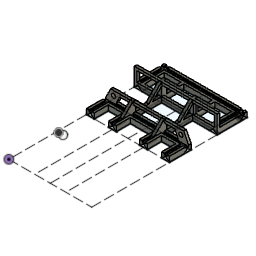
Body (1) (Autodesk Fusion 360 design; units mm, degrees)
Autodesk Fusion 360 part; units mm, degrees
sketch "스케치1" plane through (0, 0, 0) normal (0, 0, 1) x (1, 0, 0)
  line L0 (0, 0) -> (160, 0) construction
  line L1 (160, 0) -> (160, 300) construction
  line L2 (160, 300) -> (0, 300) construction
  line L3 (0, 300) -> (0, 0) construction
  line L4 (80, 0) -> (80, 300) construction
  line L5 (160, 150) -> (0, 150) construction
  line L6 (0, 192.1) -> (47.5, 192.1)
  line L7 (47.5, 192.1) -> (47.5, 242.1)
  line L8 (47.5, 242.1) -> (0, 242.1)
  line L9 (0, 242.1) -> (0, 300)
  line L10 (0, 300) -> (160, 300)
  line L11 (160, 300) -> (160, 242.1)
  line L12 (160, 242.1) -> (112.5, 242.1)
  line L13 (112.5, 242.1) -> (112.5, 192.1)
  line L14 (112.5, 192.1) -> (160, 192.1)
  line L15 (52.5, 242.1) -> (107.5, 242.1)
  line L16 (107.5, 242.1) -> (107.5, 192.1)
  line L17 (107.5, 192.1) -> (52.5, 192.1)
  line L18 (52.5, 192.1) -> (52.5, 242.1)
  line L19 (0, 247.1) -> (160, 247.1) construction
  line L20 (50, 300) -> (50, 0) construction
  line L21 (110, 300) -> (110, 0) construction
  line L22 (0, 97.8296) -> (15, 97.8296)
  line L23 (15, 97.8296) -> (15, 87.8296)
  line L24 (15, 87.8296) -> (0, 87.8296)
  line L25 (0, 87.8296) -> (0, 97.8296)
  circle A0 centre (3.4, 92.8296) radius 2
  circle A1 centre (3.4, 92.8296) radius 3.4 construction
  line L26 (6.8, 94.7926) -> (6.8, 90.8666)
  line L27 (6.8, 90.8666) -> (3.4, 88.9036)
  line L28 (3.4, 88.9036) -> (0, 90.8666)
  line L29 (0, 90.8666) -> (0, 94.7926)
  line L30 (0, 94.7926) -> (3.4, 96.7556)
  line L31 (3.4, 96.7556) -> (6.8, 94.7926)
  line L32 (0, 92.8296) -> (15, 92.8296) construction
  line L33 (15, 94.7926) -> (15, 90.8666)
  circle A2 centre (11.6, 92.8296) radius 2
  line L34 (11.6, 96.7556) -> (15, 94.7926)
  line L35 (15, 90.8666) -> (11.6, 88.9036)
  line L36 (11.6, 88.9036) -> (8.2, 90.8666)
  line L37 (8.2, 94.7926) -> (11.6, 96.7556)
  circle A3 centre (11.6, 92.8296) radius 3.4 construction
  line L38 (8.2, 90.8666) -> (8.2, 94.7926)
  line L39 (7.5, 97.8296) -> (7.5, 87.8296) construction
  line L40 (15, 242.1) -> (15, 285)
  line L41 (15, 285) -> (145, 285)
  line L42 (145, 285) -> (145, 242.1)
  line L43 (160, 247.1) -> (0, 247.1)
  line L44 (160, 192.1) -> (160, 150)
  line L45 (160, 150) -> (145, 150)
  line L46 (145, 150) -> (145, 177.1)
  line L47 (145, 177.1) -> (117.5, 177.1)
  line L48 (117.5, 177.1) -> (117.5, 150)
  line L49 (117.5, 150) -> (102.5, 150)
  line L50 (102.5, 150) -> (102.5, 177.1)
  line L51 (102.5, 177.1) -> (57.5, 177.1)
  line L52 (57.5, 177.1) -> (57.5, 150)
  line L53 (57.5, 150) -> (42.5, 150)
  line L54 (42.5, 150) -> (42.5, 177.1)
  line L55 (42.5, 177.1) -> (15, 177.1)
  line L56 (15, 177.1) -> (15, 150)
  line L57 (15, 150) -> (0, 150)
  line L58 (0, 150) -> (0, 192.1)
  circle A4 centre (152.5, 292.5) radius 1.5
  circle A5 centre (142.5, 292.5) radius 1.5
  line L59 (152.5, 291) -> (142.5, 291)
  line L60 (142.5, 294) -> (152.5, 294)
  line L61 (152.5, 292.5) -> (142.5, 292.5) construction
  dimension "d1" = 300
  dimension "d2" = 160
  dimension "d16" = 50
  dimension "d48" = 5
  dimension "d51" = 5
  dimension "d52" = 60
  dimension "d83" = 57.9
  dimension "d93" = 10
  dimension "d97" = 15
  dimension "d98" = 4
  dimension "d99" = 6.8
  dimension "d100" = 120
  dimension "d101" = 120
  dimension "d102" = 4
  dimension "d103" = 6.8
  dimension "d104" = 120
  dimension "d105" = 120
  dimension "d106" = 3.4
  dimension "d137" = 15
  dimension "d138" = 15
  dimension "d139" = 15
  dimension "d146" = 15
  dimension "d147" = 15
  dimension "d148" = 15
  dimension "d193" = 3
  dimension "d194" = 3
  dimension "d196" = 10
  dimension "d199" = 7.5
  dimension "d200" = 7.5
  constraint coincident L0.start L3.end
  constraint horizontal L0
  constraint perpendicular L0 L1
  constraint perpendicular L1 L2
  constraint perpendicular L0 L3
  constraint midpoint L0 L4.start
  constraint midpoint L2 L4.end
  constraint midpoint L1 L5.start
  constraint midpoint L3 L5.end
  constraint coincident L3 L6.start
  constraint perpendicular L6 L7
  constraint coincident L3 L8.end
  constraint perpendicular L3 L8
  constraint coincident L1 L11.end
  constraint perpendicular L1 L12
  constraint perpendicular L12 L13
  constraint coincident L1 L14.end
  constraint perpendicular L1 L14
  constraint symmetric L4 L7 L13
  constraint symmetric L4 L8 L12
  constraint symmetric L4 L6 L14
  constraint horizontal L15
  constraint vertical L16
  constraint horizontal L17
  constraint vertical L18
  constraint symmetric L4 L16 L18
  constraint coincident L3 L19.start
  constraint coincident L11 L19.end
  constraint horizontal L19
  constraint coincident L10 L20.start
  constraint coincident L0 L20.end
  constraint vertical L20
  constraint symmetric L7 L18 L20
  constraint coincident L10 L21.start
  constraint coincident L0 L21.end
  constraint perpendicular L0 L21
  constraint symmetric L13 L16 L21
  constraint collinear L12 L15
  constraint collinear L14 L17
  constraint horizontal L22
  constraint vertical L23
  constraint horizontal L24
  constraint vertical L25
  constraint coincident L3 L22.start
  constraint concentric A0 A1
  constraint vertical L26
  constraint tangent A1 L26
  constraint tangent A1 L31
  constraint tangent A1 L30
  constraint tangent A1 L27
  constraint tangent A1 L28
  constraint tangent A1 L29
  constraint vertical L29
  constraint parallel L27 L30
  constraint parallel L28 L31
  constraint midpoint L25 L32.start
  constraint midpoint L23 L32.end
  constraint concentric A2 A3
  constraint vertical L33
  constraint tangent L33 A3
  constraint tangent L34 A3
  constraint tangent L37 A3
  constraint tangent L35 A3
  constraint tangent L36 A3
  constraint tangent A3 L38
  constraint vertical L38
  constraint parallel L35 L37
  constraint parallel L34 L36
  constraint coincident A0.centre L32
  constraint midpoint L22 L39.start
  constraint midpoint L24 L39.end
  constraint symmetric A0.centre A2.centre L39
  constraint coincident L8 L40.start
  constraint perpendicular L8 L40
  constraint perpendicular L40 L41
  constraint coincident L12 L42.end
  constraint perpendicular L12 L42
  constraint coincident L5 L45.end
  constraint perpendicular L44 L45
  constraint perpendicular L45 L46
  constraint perpendicular L46 L47
  constraint coincident L5 L48.end
  constraint perpendicular L5 L48
  constraint coincident L5 L49.end
  constraint perpendicular L49 L50
  constraint perpendicular L50 L51
  constraint coincident L5 L52.end
  constraint perpendicular L5 L52
  constraint coincident L5 L53.end
  constraint perpendicular L5 L54
  constraint perpendicular L54 L55
  constraint coincident L5 L56.end
  constraint perpendicular L5 L56
  constraint perpendicular L3 L57
  constraint symmetric L20 L52 L54
  constraint symmetric L21 L48 L50
  constraint symmetric L4 L50 L52
  constraint collinear L47 L51
  constraint collinear L51 L55
  constraint coincident A4 L59.start
  constraint coincident A5 L59.end
  constraint tangent A5 L59
  constraint coincident A5 L60.start
  constraint coincident A4 L60.end
  constraint tangent A4 L60
  constraint coincident A4.centre L61.start
  constraint coincident A5.centre L61.end
  constraint parallel L59 L61
  constraint parallel L60 L61
  constraint horizontal L61
  measures "d1" distance of L0.end L1.end
  measures "d2" distance of L1.end L2.end
  measures "d16" distance of L6.end L7.end
  measures "d48" distance of L8 L19
  measures "d51" distance of L7 L18
  measures "d52" distance of L20 L21
  measures "d83" distance of L2 L8
  measures "d93" distance of L22.end L23.end
  measures "d97" distance of L22.start L22.end
  measures "d98" diameter of A0
  measures "d99" diameter of A1
  measures "d100" angle of L29 L30
  measures "d101" angle of L26 L31
  measures "d102" diameter of A2
  measures "d103" diameter of A3
  measures "d104" angle of L37 L38
  measures "d105" angle of L33 L34
  measures "d106" distance of L3 A0.centre
  measures "d137" distance of L2 L41
  measures "d138" distance of L1 L42
  measures "d139" distance of L3 L40
  measures "d146" distance of L1 L46
  measures "d147" distance of L14 L47
  measures "d148" distance of L48 L50
  measures "d193" diameter of A5
  measures "d194" diameter of A4
  measures "d196" horizontal distance of A4.centre A5.centre
  measures "d199" distance of L10 L61
  measures "d200" distance of L1 A4.centre
sketch "스케치2" plane through (0, 0, 0) normal (0, 1, 0) x (1, 0, 0)
  line L0 (0, 0) -> (160, 0)
  line L1 (160, 0) -> (160, -10)
  line L2 (160, -10) -> (150.5845, -29)
  line L3 (9.4155, -29) -> (0, -10)
  line L4 (0, -10) -> (0, 0)
  line L5 (0, -118.8837) -> (160, -118.8837) construction
  line L6 (160, -118.8837) -> (160, -153.5837)
  line L7 (160, -153.5837) -> (0, -153.5837)
  line L8 (0, -153.5837) -> (0, -118.8837)
  line L9 (80, 0) -> (80, -153.5837) construction
  line L10 (50, -153.5837) -> (50, 0) construction
  line L11 (110, -153.5837) -> (110, 0) construction
  line L12 (5, -148.5837) -> (45.7, -148.5837)
  line L13 (45.7, -148.5837) -> (45.7, -128.8837)
  line L14 (45.7, -128.8837) -> (5, -128.8837)
  line L15 (5, -128.8837) -> (5, -148.5837)
  line L16 (114.3, -148.5837) -> (155, -148.5837)
  line L17 (155, -148.5837) -> (155, -128.8837)
  line L18 (155, -128.8837) -> (114.3, -128.8837)
  line L19 (114.3, -128.8837) -> (114.3, -148.5837)
  circle A0 centre (145, -138.8837) radius 1.5
  circle A1 centre (15, -138.8837) radius 1.5
  circle A2 centre (15, -20) radius 4
  circle A3 centre (145, -20) radius 4
  line L20 (15, -138.8837) -> (15, -20) construction
  line L21 (145, -138.8837) -> (145, -20) construction
  line L22 (9.4155, -29) -> (150.5845, -29)
  line L23 (27.0267, -24) -> (47.5, -24)
  line L24 (47.5, -24) -> (47.5, -10)
  line L25 (47.5, -10) -> (20.0889, -10)
  line L26 (20.0889, -10) -> (27.0267, -24)
  line L27 (112.5, -24) -> (112.5, -10)
  line L28 (112.5, -10) -> (139.9111, -10)
  line L29 (139.9111, -10) -> (132.9733, -24)
  line L30 (132.9733, -24) -> (112.5, -24)
  line L31 (52.5, -24) -> (107.5, -24)
  line L32 (107.5, -24) -> (107.5, -10)
  line L33 (107.5, -10) -> (52.5, -10)
  line L34 (52.5, -10) -> (52.5, -24)
  line L35 (52.5, -148.5837) -> (107.5, -148.5837)
  line L36 (107.5, -148.5837) -> (107.5, -128.8837)
  line L37 (107.5, -128.8837) -> (52.5, -128.8837)
  line L38 (52.5, -128.8837) -> (52.5, -148.5837)
  line L39 (0, 0) -> (160, 0)
  line L40 (160, -118.8837) -> (158.5, -118.8837)
  line L41 (158.5, -118.8837) -> (152.5, -124.8837)
  line L42 (152.5, -124.8837) -> (146.5, -118.8837)
  line L43 (152.5, -124.8837) -> (152.5, -122.5068) construction
  line L44 (0, -118.8837) -> (1.5, -118.8837)
  line L45 (1.5, -118.8837) -> (7.5, -124.8837)
  line L46 (7.5, -124.8837) -> (13.5, -118.8837)
  line L47 (13.5, -118.8837) -> (146.5, -118.8837)
  line L48 (145, -20) -> (15, -20)
  circle A4 centre (15, -20) radius 1.5
  circle A5 centre (145, -20) radius 1.5
  dimension "d50" = 160
  dimension "d53" = 60
  dimension "d54" = 10
  dimension "d58" = 5
  dimension "d59" = 5
  dimension "d61" = 3
  dimension "d69" = 10
  dimension "d70" = 10
  dimension "d71" = 40.7
  dimension "d72" = 19.7
  dimension "d73" = 10
  dimension "d74" = 8
  dimension "d75" = 20
  dimension "d76" = 9
  dimension "d77" = 9
  dimension "d78" = 5
  dimension "d79" = 9
  dimension "d80" = 5
  dimension "d82" = 10
  dimension "d133" = 45
  dimension "d134" = 1.5
  dimension "d136" = 7.5
  dimension "d145" = 3
  constraint coincident L0.start L4.end
  constraint horizontal L0
  constraint perpendicular L0 L1
  constraint perpendicular L4 L5
  constraint perpendicular L5 L6
  constraint perpendicular L6 L7
  constraint perpendicular L5 L8
  constraint collinear L4 L8
  constraint collinear L1 L6
  constraint midpoint L0 L9.start
  constraint midpoint L7 L9.end
  constraint coincident L7 L10.start
  constraint coincident L0 L10.end
  constraint coincident L7 L11.start
  constraint coincident L0 L11.end
  constraint perpendicular L0 L11
  constraint symmetric L2 L3 L9
  constraint horizontal L12
  constraint vertical L13
  constraint horizontal L14
  constraint vertical L15
  constraint horizontal L16
  constraint vertical L17
  constraint horizontal L18
  constraint vertical L19
  constraint symmetric L9 L13 L19
  constraint symmetric L9 L15 L17
  constraint collinear L12 L16
  constraint collinear L14 L18
  constraint symmetric L9 A0 A1
  constraint symmetric L9 A2 A3
  constraint coincident A1.centre L20.start
  constraint coincident A2.centre L20.end
  constraint coincident A0.centre L21.start
  constraint coincident A3.centre L21.end
  constraint vertical L21
  constraint perpendicular L20 L22
  constraint perpendicular L10 L23
  constraint perpendicular L23 L24
  constraint perpendicular L10 L25
  constraint perpendicular L23 L27
  constraint perpendicular L27 L28
  constraint perpendicular L27 L30
  constraint perpendicular L9 L31
  constraint perpendicular L31 L32
  constraint perpendicular L9 L33
  constraint vertical L34
  constraint parallel L3 L26
  constraint collinear L23 L31
  constraint collinear L30 L31
  constraint collinear L28 L33
  constraint collinear L25 L33
  constraint symmetric L9 L26 L29
  constraint symmetric L9 L24 L27
  constraint symmetric L11 L27 L32
  constraint perpendicular L9 L35
  constraint perpendicular L7 L36
  constraint perpendicular L36 L37
  constraint vertical L38
  constraint collinear L34 L38
  constraint collinear L32 L36
  constraint collinear L18 L37
  constraint collinear L16 L35
  constraint coincident L5 L40.end
  constraint coincident L5 L42.end
  constraint perpendicular L41 L42
  constraint vertical L43
  constraint coincident L5 L44.end
  constraint coincident L5 L46.end
  constraint perpendicular L45 L46
  constraint symmetric L9 L41 L45
  constraint symmetric L9 L42 L46
  constraint equal A4 A5
  measures "d50" distance of L0.start L0.end
  measures "d53" distance of L10 L11
  measures "d54" distance of L3.end L0.start
  measures "d58" distance of L8 L15
  measures "d59" distance of L7 L12
  measures "d61" diameter of A0
  measures "d69" distance of L17 A0.centre
  measures "d70" distance of L18 A0.centre
  measures "d71" distance of L12.start L12.end
  measures "d72" distance of L12.start L14.end
  measures "d73" distance of L5 L14
  measures "d74" diameter of A2
  measures "d75" distance of L0 A2.centre
  measures "d76" distance of A2.centre L22
  measures "d77" distance of L3 A2.centre
  measures "d78" distance of L22 L31
  measures "d79" distance of A2.centre L26
  measures "d80" distance of L27 L32
  measures "d82" distance of L33 L39
  measures "d133" angle of L5 L41
  measures "d134" distance of L5.end L40.end
  measures "d136" distance of L6 L43
  measures "d145" diameter of A4
sketch "스케치4" plane through (0, 0, 0) normal (1, 0, 0) x (0, 1, 0)
  line L0 (0, 0) -> (300, 0) construction
  line L1 (150, 0) -> (150, 280) construction
  line L2 (300, 0) -> (300, 10)
  line L3 (242.1, 0) -> (242.1, 34.7)
  line L4 (242.1, 34.7) -> (252.1, 34.7)
  line L5 (192.1, 0) -> (192.1, 29.6923)
  line L6 (150, 10) -> (150, 0)
  line L7 (300, 10) -> (150, 10) construction
  line L8 (192.1, 0) -> (150, 0)
  line L9 (252.1, 34.7) -> (276.8, 10)
  line L10 (269.7289, 10) -> (252.1, 10)
  line L11 (252.1, 10) -> (252.1, 27.6289)
  line L12 (252.1, 27.6289) -> (269.7289, 10)
  line L13 (167.5749, 10) -> (187.1, 29.6923)
  line L14 (187.1, 29.6923) -> (192.1, 29.6923)
  line L15 (242.1, 34.7) -> (217.4, 10)
  line L16 (192.1, 29.6923) -> (211.7923, 10)
  line L17 (224.4711, 10) -> (242.1, 27.6289)
  line L18 (192.1, 22.6212) -> (204.7212, 10)
  line L19 (242.1, 10) -> (192.1, 10)
  line L20 (300, 0) -> (298.5, 0)
  line L21 (298.5, 0) -> (292.5, 6)
  line L22 (292.5, 6) -> (286.5, 0)
  line L23 (286.5, 0) -> (242.1, 0)
  line L24 (300, 10) -> (295.2, 10)
  line L25 (295.2, 10) -> (295.2, 7.5)
  line L26 (295.2, 7.5) -> (289.8, 7.5)
  line L27 (289.8, 7.5) -> (289.8, 10)
  line L28 (289.8, 10) -> (276.8, 10)
  line L29 (292.5, 7.5) -> (292.5, 6) construction
  line L30 (242.1, 0) -> (192.1, 0)
  line L31 (70, 135) -> (82, 135)
  line L32 (82, 135) -> (76, 141)
  line L33 (76, 141) -> (70, 135)
  line L34 (75.6, 152.5) -> (81, 152.5)
  line L35 (81, 152.5) -> (81, 155)
  line L36 (81, 155) -> (75.6, 155)
  line L37 (75.6, 155) -> (75.6, 152.5)
  line L38 (286.5, 0) -> (298.5, 0)
  line L39 (289.8, 10) -> (295.2, 10)
  line L40 (150, 7.5) -> (165.0749, 7.5)
  line L41 (165.0749, 7.5) -> (167.5749, 10)
  dimension "d111" = 300
  dimension "d112" = 57.9
  dimension "d113" = 50
  dimension "d115" = 34.7
  dimension "d116" = 10
  dimension "d121" = 10
  dimension "d122" = 135
  dimension "d123" = 10
  dimension "d124" = 5
  dimension "d126" = 5
  dimension "d129" = 45
  dimension "d130" = 45
  dimension "d131" = 5
  dimension "d132" = 5
  dimension "d140" = 45
  dimension "d141" = 1.5
  dimension "d142" = 7.5
  dimension "d143" = 2.5
  dimension "d144" = 5.4
  dimension "d157" = 12
  dimension "d158" = 45
  dimension "d159" = 45
  dimension "d160" = 5.4
  dimension "d161" = 2.5
  dimension "d181" = 2.5
  dimension "d184" = 135
  constraint coincident L0.start origin
  constraint horizontal L0
  constraint midpoint L0 L1.start
  constraint perpendicular L0 L1
  constraint perpendicular L0 L2
  constraint coincident L0 L3.start
  constraint perpendicular L0 L3
  constraint coincident L0 L5.start
  constraint perpendicular L0 L5
  constraint coincident L0 L1.start
  constraint perpendicular L0 L6
  constraint horizontal L4
  constraint coincident L1 L6.start
  constraint perpendicular L1 L7
  constraint coincident L7 L9.end
  constraint coincident L7 L10.start
  constraint coincident L7 L10.end
  constraint perpendicular L10 L11
  constraint parallel L9 L12
  constraint coincident L6.start L7
  constraint coincident L7 L13.start
  constraint horizontal L14
  constraint coincident L7 L15.end
  constraint coincident L7 L16.end
  constraint coincident L7 L17.start
  constraint coincident L3 L17.end
  constraint parallel L15 L17
  constraint coincident L5 L18.start
  constraint coincident L7 L18.end
  constraint perpendicular L17 L18
  constraint coincident L7 L19.start
  constraint coincident L3 L19.start
  constraint coincident L7 L19.end
  constraint coincident L5 L19.end
  constraint coincident L0 L20.end
  constraint coincident L0 L22.end
  constraint perpendicular L21 L22
  constraint coincident L7 L24.end
  constraint perpendicular L7 L25
  constraint perpendicular L25 L26
  constraint coincident L7 L27.end
  constraint perpendicular L7 L27
  constraint midpoint L26 L29.start
  constraint vertical L29
  constraint collinear L1 L6
  constraint horizontal L31
  constraint parallel L31 L34
  constraint perpendicular L31 L35
  constraint perpendicular L35 L36
  constraint perpendicular L36 L37
  constraint coincident L6 L40.start
  constraint perpendicular L6 L40
  measures "d111" distance of L0.start L0.end
  measures "d112" distance of L2 L3
  measures "d113" distance of L3 L5
  measures "d115" distance of L3.start L3.end
  measures "d116" distance of L0.end L2.end
  measures "d121" distance of L4.end L3.end
  measures "d122" angle of L7 L9
  measures "d123" distance of L3 L11
  measures "d124" distance of L9 L12
  measures "d126" distance of L5.end L13.end
  measures "d129" angle of L5 L16
  measures "d130" angle of L3 L15
  measures "d131" distance of L16 L18
  measures "d132" distance of L15 L17
  measures "d140" angle of L0 L21
  measures "d141" distance of L0.end L20.end
  measures "d142" distance of L2 L29
  measures "d143" distance of L24.end L25.end
  measures "d144" distance of L25.end L26.end
  measures "d157" distance of L31.start L31.end
  measures "d158" angle of L31 L32
  measures "d159" angle of L31 L33
  measures "d160" distance of L35.end L36.end
  measures "d161" distance of L34.end L35.end
  measures "d181" distance of L7 L40
  measures "d184" angle of L40 L41
extrude "돌출1" add sketch "스케치1" along normal blind 10 contours L6 L7 L8 L12 L13 L14 L40 L42 L43 L44 L45 L46 L47 L48 L49 L50 L51 L52 L53 L54 L55 L56 L57 L58 | L8 L9 L40 L43 | L9 L10 L11 L40 L41 L42 L43 | L11 L12 L42 L43 | A4 | A4 A5 L59 L60 | A5 makes body 1
extrude "돌출5" add sketch "스케치4" along normal blind 350 separate body contours L31 L32 L33 makes body 2
move_body "정렬5" bodies 2 to x (1, 0, 0) y (0, 1, 0) z (0, 0, 1) at (0, 110.1, -135)
move_body "이동2" bodies 2 to x (1, 0, 0) y (0, 1, 0) z (0, 0, 1) at (0, -1.5, 0)
combine "결합5" operation cut target body 1 tool bodies 2
extrude "돌출6" cut sketch "스케치4" along normal blind 200 contours L21 L22 L38 bodies 1
extrude "돌출7" cut sketch "스케치4" along normal blind 180 contours L25 L26 L27 L39 bodies 1
extrude "돌출8" add sketch "스케치4" along normal blind 290 separate body contours L34 L35 L36 L37 makes body 3
move_body "정렬6" bodies 3 to x (1, 0, 0) y (0, 1, 0) z (0, 0, 1) at (-130, 111.1, -145)
move_body "이동3" bodies 3 to x (1, 0, 0) y (0, 1, 0) z (0, 0, 1) at (0, -4.8, 0)
combine "결합6" operation cut target body 1 tool bodies 3
extrude "돌출9" add sketch "스케치4" along normal blind 250 separate body contours L31 L32 L33 makes body 4
move_body "정렬7" bodies 4 to x (0, 1, 0) y (-1, 0, 0) z (0, 0, 1) at (83.5, 150, -135)
combine "결합7" operation cut target body 1 tool bodies 4
extrude "돌출10" add sketch "스케치4" along normal blind 240 separate body contours L34 L35 L36 L37 makes body 5
move_body "정렬8" bodies 5 to x (0, 1, 0) y (-1, 0, 0) z (0, 0, 1) at (85.8, 150, -145)
combine "결합8" operation cut target body 1 tool bodies 5
extrude "돌출11" add sketch "스케치4" along normal blind 34.6 separate body contours L31 L32 L33 | L34 L35 L36 L37 makes body 6 at (23.0667, 74, 135) makes body 7 at (11.5333, 79.2, 155)
move_body "정렬9" bodies 6 to x (0, 1, 0) y (-1, 0, 0) z (0, 0, 1) at (126, 150, -135)
combine "결합9" operation cut target body 1 tool bodies 6
move_body "정렬10" bodies 7 to x (0, 1, 0) y (-1, 0, 0) z (0, 0, 1) at (128.3, 150, -145)
combine "결합10" operation cut target body 1 tool bodies 7
extrude "돌출12" add sketch "스케치4" along normal blind 34.6 separate body contours L31 L32 L33 | L34 L35 L36 L37 makes body 8 at (23.0667, 74, 135) makes body 9 at (11.5333, 79.2, 155)
move_body "정렬11" bodies 8 to x (0, 1, 0) y (-1, 0, 0) z (0, 0, 1) at (186, 150, -135)
move_body "정렬12" bodies 9 to x (0, 1, 0) y (-1, 0, 0) z (0, 0, 1) at (188.3, 150, -145)
combine "결합11" operation cut target body 1 tool bodies 8
combine "결합12" operation cut target body 1 tool bodies 9
extrude "돌출13" add sketch "스케치4" along normal blind 250 separate body contours L31 L32 L33 | L34 L35 L36 L37 makes body 10 at (83.3333, 79.2, 155) makes body 11 at (83.3333, 74, 135)
move_body "정렬13" bodies 10 to x (0, 1, 0) y (-1, 0, 0) z (0, 0, 1) at (230.8, 150, -145)
move_body "정렬14" bodies 11 to x (0, 1, 0) y (-1, 0, 0) z (0, 0, 1) at (228.5, 150, -135)
combine "결합13" operation cut target body 1 tool bodies 10
combine "결합14" operation cut target body 1 tool bodies 11
extrude "돌출14" add sketch "스케치4" along normal blind 5.4 separate body contours L2 L3 L4 L9 L20 L21 L22 L23 L24 L25 L26 L27 L28 | L3 L5 L19 L30 | L5 L6 L8 L13 L14 L40 L41 | L3 L15 L17 L19 | L5 L16 L18 L19 makes body 12
copy_body "CopyPasteBodies2" bodies 12 makes body 13
move_body "이동4" bodies 13 to x (1, 0, 0) y (0, 1, 0) z (0, 0, 1) at (60, 0, 0)
move_body "정렬15" bodies 12 to x (1, 0, 0) y (0, 1, 0) z (0, 0, 1) at (47.3, 0, 0)
move_body "정렬16" bodies 13 to x (1, 0, 0) y (0, 1, 0) z (0, 0, 1) at (47.3, 0, 0)
combine "결합15" operation add target body 13 tool bodies 1
combine "결합16" operation add target body 12 tool bodies 13
extrude "돌출15" add sketch "스케치2" along normal blind 5 separate body contours L6 L7 L8 L40 L41 L42 L44 L45 L46 L47 makes body 14
move_body "정렬17" bodies 14 to x (1, 0, 0) y (0, 1, 0) z (0, 0, 1) at (0, 242.1, -118.8837)
extrude "돌출16" add sketch "스케치2" along normal blind 5 separate body contours L0 L1 L2 L3 L4 L22 L39 makes body 15
move_body "정렬18" bodies 15 to x (1, 0, 0) y (0, 1, 0) z (0, 0, 1) at (0, 187.1, 0)
combine "결합17" operation add target body 14 tool bodies 12
combine "결합18" operation add target body 14 tool bodies 15
extrude "돌출17" add sketch "스케치4" along normal blind 34.6 separate body contours L31 L32 L33 makes body 16
copy_body "CopyPasteBodies3" bodies 16 makes body 17
move_body "이동5" bodies 17 to x (1, 0, 0) y (0, 1, 0) z (0, 0, 1) at (0, 25, 0)
move_body "정렬19" bodies 17 to x (0, -1, 0) y (1, 0, 0) z (0, 0, 1) at (-51, 184.6, -135)
move_body "정렬20" bodies 16 to x (0, -1, 0) y (1, 0, 0) z (0, 0, 1) at (34, 184.6, -135)
combine "결합19" operation cut target body 14 tool bodies 16
combine "결합20" operation cut target body 14 tool bodies 17
extrude "돌출18" add sketch "스케치4" along normal blind 180 separate body contours L31 L32 L33 makes body 18
move_body "정렬21" bodies 18 to x (1, 0, 0) y (0, 1, 0) z (0, 0, 1) at (0, 108.6, -135)
combine "결합21" operation cut target body 14 tool bodies 18
extrude "돌출19" add sketch "스케치1" along normal blind 10 separate body contours A4 | A4 A5 L59 L60 | A5 makes body 19
pattern_linear "R-패턴2" count 7 spacing 20 along (-1, 0, 0) of bodies 19 makes body 20 at (125.8333, 294, 3.3333) makes body 21 at (105.8333, 294, 3.3333) makes body 22 at (85.8333, 294, 3.3333) makes body 23 at (65.8333, 294, 3.3333) makes body 24 at (45.8333, 294, 3.3333) makes body 25 at (25.8333, 294, 3.3333)
combine "결합23" operation cut target body 14 tool bodies 19
combine "결합24" operation cut target body 14 tool bodies 20
combine "결합25" operation cut target body 14 tool bodies 21
combine "결합26" operation cut target body 14 tool bodies 22
combine "결합27" operation cut target body 14 tool bodies 23
combine "결합28" operation cut target body 14 tool bodies 24
equation "m3hole = 3 mm" comment "m3 볼트 스크류 크기"
equation "m3width = 5.4 mm" comment "m3너트 크기"
equation "m3height = 2.5 mm" comment "m3너트 높이"
equation "frame = 15 mm" comment "레일 너비"
equation "thk = 10 mm" comment "뼈대 너비"
equation "thn = 5 mm"
equation "error = 0.4 mm" comment "공차"
equation "d48 = thn"
equation "d50 = d2"
equation "d51 = thn"
equation "d53 = d52"
equation "d54 = thk"
equation "d58 = thn"
equation "d59 = thn"
equation "bearing_height = 4 mm"
equation "bearing_out = 8 mm" comment "베어링 밖쪽 반지름"
equation "bearing_in = 3 mm" comment "베어링 안쪽 반지름"
equation "moter_len = 19.7 mm"
equation "moter_wid = 40.7 mm"
equation "moter_hole_len = 10 mm"
equation "moter_hole_wid = 10 mm"
equation "d69 = moter_hole_wid"
equation "d70 = moter_hole_len"
equation "d71 = moter_wid"
equation "d72 = moter_len"
equation "d73 = d54"
equation "d74 = bearing_out"
equation "d75 = d73 + d70"
equation "d76 = bearing_out / 2 + thn"
equation "d77 = d76"
equation "d78 = thn"
equation "d79 = d76"
equation "d80 = d51"
equation "d82 = d54"
equation "d83 = moter_height + frame"
equation "moter_height = 42.9 mm"
equation "d93 = d54"
equation "m4_width = 6.8 mm"
equation "m4_hole = 4 mm"
equation "m4_height = 3 mm"
equation "d97 = frame"
equation "d98 = m4_hole"
equation "d99 = m4_width"
equation "d102 = m4_hole"
equation "d103 = m4_width"
equation "d106 = m4_width / 2"
equation "d111 = d1"
equation "d112 = d83"
equation "d113 = d16"
equation "d115 = d73 + d72 + d59"
equation "d116 = d54"
equation "d121 = thk"
equation "d123 = d121"
equation "d124 = thn"
equation "d126 = thn"
equation "d131 = thn"
equation "d132 = thn"
equation "d137 = frame"
equation "d138 = frame"
equation "d139 = frame"
equation "d143 = m3height"
equation "d144 = m3width"
equation "d145 = bearing_in"
equation "d146 = frame"
equation "d147 = frame"
equation "d148 = frame"
equation "d149 = thk"
equation "d160 = m3width"
equation "d161 = m3height"
equation "d174 = 42.1 mm - 7.5 mm"
equation "d176 = 42.1 mm - 7.5 mm"
equation "d181 = m3height"
equation "d189 = 42.1 mm - 7.5 mm"
equation "d193 = m3hole"
equation "d194 = m3hole"
equation "d199 = frame / 2"
equation "d200 = frame / 2"
